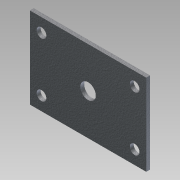
# Autodesk Inventor part: mount plate
Saved by Autodesk Inventor 2012 (Build 160160000, 160)
## iProperties
Created: 2012-09-15
Part Number: mount plate
Material: Default
Document SubType Name: Modeling
Designer: Admin
Density: 1 g/cm^3
Author: Admin
Autodesk Inventor part; units mm, degrees
ref_plane "YZ Plane" through (0, 0, 0) normal (1, 0, 0) x (0, 1, 0)
ref_plane "XZ Plane" through (0, 0, 0) normal (0, 1, 0) x (-1, 0, 0)
ref_plane "XY Plane" through (0, 0, 0) normal (0, 0, 1) x (1, 0, 0)
sketch "Sketch1" plane through (0, 0, 0) normal (0, 0, 1) x (1, 0, 0)
  line L0 (0, 0) -> (-95.25, 0)
  line L1 (-95.25, 0) -> (-95.25, 66.675)
  line L2 (-95.25, 66.675) -> (0, 66.675)
  line L3 (0, 66.675) -> (0, 0)
  dimension "d0" = 66.675
  dimension "d1" = 95.25
  constraints: 8 end point, 2 parallel, 1 horizontal, 1 perpendicular
  measures "d0" distance of L2.end L0.start
  measures "d1" distance of L0.start L0.end
extrude "Extrusion1" add sketch "Sketch1" along normal blind 3.175
sketch "Sketch2" plane through (0, 0, 3.175) normal (0, 0, 1) x (1, 0, 0)
  line L0 (-95.25, 0) -> (-95.25, 66.675) projected
  line L1 (0, 66.675) -> (0, 0) projected
  line L2 (-95.25, 66.675) -> (0, 66.675) projected
  line L3 (-95.25, 33.3375) -> (-95.25, 55.5625)
  line L4 (-47.625, 66.675) -> (-85.725, 66.675)
  line L5 (-85.725, 66.675) -> (-85.725, 55.5625)
  line L6 (-95.25, 33.3375) -> (-95.25, 11.1125)
  line L7 (-95.25, 11.1125) -> (-85.725, 11.1125)
  line L8 (-47.625, 66.675) -> (-9.525, 66.675)
  line L9 (-9.525, 66.675) -> (-9.525, 55.5625)
  line L10 (0, 11.1125) -> (-9.525, 11.1125)
  circle A0 centre (-85.725, 55.5625) radius 3.9687
  circle A1 centre (-9.525, 55.5625) radius 3.9688
  circle A2 centre (-85.725, 11.1125) radius 3.9688
  circle A3 centre (-9.525, 11.1125) radius 3.9688
  dimension "d4" = 22.225
  dimension "d5" = 38.1
  dimension "d6" = 22.225
  dimension "d7" = 38.1
  dimension "d8" = 7.9375
  dimension "d9" = 7.9375
  dimension "d10" = 7.9375
  dimension "d11" = 7.9375
  constraints: 16 end point, 5 point on line, 4 centre point, 4 coincident, 4 perpendicular, 2 midpoint
  measures "d4" distance of L3.start L3.end
  measures "d5" distance of L4.start L4.end
  measures "d6" distance of L3.start L6.end
  measures "d7" distance of L4.start L8.end
  measures "d8" diameter of A0
  measures "d9" diameter of A1
  measures "d10" diameter of A2
  measures "d11" diameter of A3
extrude "Extrusion2" cut sketch "Sketch2" against normal blind 3.175
sketch "Sketch3" plane through (0, 0, 3.175) normal (0, 0, 1) x (1, 0, 0)
  circle A0 centre (-47.625, 33.3375) radius 6.35
  dimension "d14" = 12.7
  constraints: 1 centre point
  measures "d14" diameter of A0
extrude "Extrusion3" cut sketch "Sketch3" against normal blind 3.175
body "Solid1"
